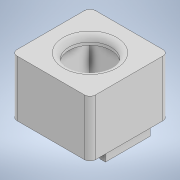
# Autodesk Inventor part: Small_Button_Part_Two
Saved by Autodesk Inventor 2021 (Build 250183000, 183)
## iProperties
Created: 2020-06-01
Part Number: Small_Button_Part_Two
Material: Generic
Document SubType Name: Modeling
Designer: ameli
Density: 1 g/cm^3
Appearance: Default
Author: ameli
Autodesk Inventor part; units mm, degrees
ref_plane "YZ Plane" through (0, 0, 0) normal (1, 0, 0) x (0, 1, 0)
ref_plane "XZ Plane" through (0, 0, 0) normal (0, 1, 0) x (-1, 0, 0)
ref_plane "XY Plane" through (0, 0, 0) normal (0, 0, 1) x (1, 0, 0)
sketch "Sketch1" plane through (0, 0, 0) normal (0, 1, 0) x (-1, 0, 0)
  line L0 (0, 0) -> (14, 0)
  line L1 (14, 0) -> (14, -14)
  line L2 (14, -14) -> (0, -14)
  line L3 (0, -14) -> (0, 0)
  dimension "d0" = 14
  dimension "d1" = 14
  constraints: 8 end point, 2 parallel, 1 horizontal, 1 perpendicular
  measures "d0" distance of L1.end L2.end
  measures "d1" distance of L0.end L1.end
extrude "Extrusion1" add sketch "Sketch1" along normal blind 10
fillet "Fillet2" radius 1 4 edges at (0, 5, 0) (0, 5, -14) (-14, 5, 0) (-14, 5, -14)
shell "Shell1" thickness 1.5 removed faces 1 at (-9.3333, 0, -9)
sketch "Sketch2" plane through (0, 10, 0) normal (0, 1, 0) x (1, 0, 0)
  circle A0 centre (-7, 7) radius 3.75
  line L0 (-1, 14) -> (-13, 14) projected
  line L1 (-14, 13) -> (-14, 1) projected
  point P0 (0, 0)
  dimension "d7" = 7.5
  dimension "d8" = 7
  dimension "d9" = 7
  constraints: 1 centre point
  measures "d7" diameter of A0
  measures "d8" distance from line of L0 A0.centre
  measures "d9" distance from line of A0.centre L1
extrude "Extrusion2" cut sketch "Sketch2" along normal mid plane 8.532
fillet "Fillet3" radius 1 1 edges at (-10.75, 10, -7)
sketch "Sketch3" plane through (0, 0, 0) normal (0, -1, 0) x (1, 0, 0)
  line L0 (-0.25, -11) -> (-1.25, -11)
  line L1 (-1.25, -11) -> (-1.25, -3)
  line L2 (-1.25, -3) -> (-0.25, -3)
  line L3 (-0.25, -3) -> (-0.25, -11)
  line L4 (0, -1) -> (0, -13) projected
  line L5 (-13, 0) -> (-1, 0) projected
  line L6 (-12.75, -11) -> (-13.75, -11)
  line L7 (-13.75, -11) -> (-13.75, -3)
  line L8 (-13.75, -3) -> (-12.75, -3)
  line L9 (-12.75, -3) -> (-12.75, -11)
  line L10 (-14, -13) -> (-14, -1) projected
  point P0 (0, 0)
  dimension "d13" = 8
  dimension "d14" = 1
  dimension "d15" = 0.25
  dimension "d16" = 3
  dimension "d17" = 1
  dimension "d18" = 8
  dimension "d19" = 0.25
  dimension "d20" = 3
  constraints: 16 end point, 4 parallel, 2 horizontal, 2 perpendicular
  measures "d13" distance of L0.end L1.end
  measures "d14" distance of L1.end L2.end
  measures "d15" distance between parallel lines of L4 L3
  measures "d16" distance between parallel lines of L5 L2
  measures "d17" distance of L6.start L6.end
  measures "d18" distance of L6.end L7.end
  measures "d19" distance between parallel lines of L10 L7
  measures "d20" distance between parallel lines of L5 L8
extrude "Extrusion3" add sketch "Sketch3" along normal blind 1.5
body "Solid1"
